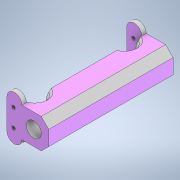
# Autodesk Inventor part: rollerbase(v2)
Saved by Autodesk Inventor 2022 (Build 260153000, 153)
## iProperties
Created: 2022-10-27
Part Number: rollerbase(v2)
Material: Generic
Document SubType Name: Modeling
Designer: matia
Density: 1 g/cm^3
Appearance: Default
Author: matia
Autodesk Inventor part; units mm, degrees
ref_plane "YZ Plane" through (0, 0, 0) normal (1, 0, 0) x (0, 1, 0)
ref_plane "XZ Plane" through (0, 0, 0) normal (0, 1, 0) x (-1, 0, 0)
ref_plane "XY Plane" through (0, 0, 0) normal (0, 0, 1) x (1, 0, 0)
sketch "Sketch1" plane through (0, 0, 0) normal (0, 1, 0) x (-1, 0, 0)
  line L0 (0, -3.556) -> (0, -34.544)
  arc A0 (0, 3.556) -> (0, -3.556) centre (0, 0) ccw
  arc A1 (0, -34.544) -> (0, -41.656) centre (0, -38.1) ccw
  line L1 (0, 3.556) -> (0, 5.461)
  line L2 (0, -41.656) -> (0, -43.561)
  line L3 (0, 7.366) -> (-13.335, 7.366)
  line L4 (0, -45.466) -> (-13.335, -45.466)
  line L5 (-13.335, -45.466) -> (-13.335, 7.366)
  line L6 (0, 7.366) -> (3.175, 7.366)
  line L7 (3.175, 5.461) -> (0, 5.461)
  line L8 (0, -45.466) -> (3.175, -45.466)
  line L9 (3.175, -43.561) -> (0, -43.561)
  line L10 (3.175, 7.366) -> (4.445, 7.366)
  line L11 (4.445, 7.366) -> (4.445, 5.461)
  line L12 (4.445, 5.461) -> (3.175, 5.461)
  line L13 (3.175, -43.561) -> (4.445, -43.561)
  line L14 (4.445, -43.561) -> (4.445, -45.466)
  line L15 (4.445, -45.466) -> (3.175, -45.466)
  dimension "d1" = 7.112
  constraints: 32 end point, 4 horizontal, 4 perpendicular, 4 point on circle, 3 vertical, 2 centre point, 2 parallel, 2 point on line, 1 coincident
  measures "d1" diameter of A0
extrude "Extrusion1" add sketch "Sketch1" along normal blind 12.7
sketch "Sketch2" plane through (13.335, 0, -45.466) normal (0, 0, -1) x (-1, 0, 0)
  line L0 (13.335, 0) -> (17.78, 0) projected
  line L1 (13.335, 0) -> (15.5575, 0)
  line L2 (17.78, 0) -> (17.78, 12.7) projected
  line L3 (17.78, 6.35) -> (15.5575, 6.35)
  line L4 (15.5575, 6.35) -> (15.5575, 0)
  line L5 (15.5575, 6.35) -> (15.5575, 3.81)
  circle A0 centre (15.5575, 3.81) radius 1.5875
  line L6 (15.5575, 6.35) -> (15.5575, 8.89)
  circle A1 centre (15.5575, 8.89) radius 1.5875
  dimension "d10" = 2.54
  dimension "d11" = 3.175
  dimension "d12" = 2.54
  dimension "d13" = 3.175
  constraints: 10 end point, 2 centre point, 2 coincident, 2 midpoint, 1 horizontal, 1 perpendicular, 1 point on line, 1 vertical
  measures "d10" distance of L3.end L5.end
  measures "d11" diameter of A0
  measures "d12" distance of L3.end L6.end
  measures "d13" diameter of A1
extrude "Extrusion2" cut sketch "Sketch2" against normal through all contours A0 L4 | L4 A0 | A1
sketch "Sketch3" plane through (0, 12.7, 0) normal (0, 1, 0) x (1, 0, 0)
  line L0 (0, -5.461) -> (1.905, -5.461)
  line L1 (1.905, -5.461) -> (1.905, 43.561)
  line L2 (1.905, 43.561) -> (0, 43.561)
  line L3 (0, 43.561) -> (0, -5.461)
  point P0 (0, 0)
  dimension "d16" = 1.905
  constraints: 8 end point, 2 parallel, 1 horizontal, 1 perpendicular
  measures "d16" distance of L2.end L1.end
extrude "Extrusion3" cut sketch "Sketch3" against normal through all
chamfer "Chamfer1" distance 3.175 angle 45 2 edges at (13.335, 12.7, -19.05) (13.335, 0, -19.05)
chamfer "Chamfer2" distance 1.905 angle 45 4 edges at (3.556, 0, -38.1) (3.556, 0, 0) (3.556, 12.7, 0) (3.556, 12.7, -38.1)
fillet "Fillet1" radius 3.175 4 edges at (3.556, 1.905, -38.1) (3.556, 10.795, -38.1) (3.556, 1.905, 0) (3.556, 10.795, 0)
sketch "Sketch4" plane through (-4.445, 0, 7.366) normal (0, 0, 1) x (1, 0, 0)
  line L0 (17.78, 3.175) -> (17.78, 9.525) projected
  line L1 (17.78, 6.35) -> (10.16, 6.35)
  line L2 (17.78, 6.35) -> (11.43, 6.35)
  circle A0 centre (11.43, 6.35) radius 3.175
  point P0 (4.445, 0)
  dimension "d26" = 7.62
  dimension "d27" = 6.35
  dimension "d28" = 6.35
  constraints: 4 end point, 1 centre point, 1 coincident, 1 horizontal, 1 midpoint, 1 point on line
  measures "d26" distance of L1.start L1.end
  measures "d27" distance of L1.start L2.end
  measures "d28" diameter of A0
extrude "Extrusion4" cut sketch "Sketch4" against normal blind 12.7
sketch "Sketch5" plane through (-4.445, 0, -45.466) normal (0, 0, -1) x (-1, 0, 0)
  line L0 (-17.78, 3.175) -> (-17.78, 9.525) projected
  line L1 (-17.78, 6.35) -> (-11.43, 6.35)
  circle A0 centre (-11.43, 6.35) radius 3.175
  point P0 (-4.445, 0)
  dimension "d31" = 6.35
  constraints: 2 end point, 1 centre point, 1 coincident, 1 horizontal, 1 midpoint
  measures "d31" distance of L1.start L1.end
extrude "Extrusion5" cut sketch "Sketch5" against normal blind 12.7
sketch "Sketch6" plane through (-4.445, 0, -43.561) normal (0, 0, 1) x (1, 0, 0)
  line L0 (0, 12.7) -> (6.35, 12.7) projected
  line L1 (6.35, 12.7) -> (6.35, 0)
  line L2 (0, 0) -> (6.35, 0) projected
  line L3 (6.35, 0) -> (0, 0)
  line L4 (0, 0) -> (0, 12.7)
  point P0 (4.445, 0)
  constraints: 6 end point, 2 perpendicular, 1 vertical
sketch "Sketch7" plane through (0, 12.7, 0) normal (0, 1, 0) x (1, 0, 0)
  line L0 (-4.445, 43.561) -> (1.905, 43.561) projected
  line L1 (-4.445, 45.466) -> (-4.445, 43.561) projected
  line L2 (-4.445, 43.561) -> (-4.445, 45.466)
  line L3 (-4.445, 43.561) -> (1.905, 43.561)
  line L4 (10.16, 45.466) -> (-4.445, 45.466) projected
  line L5 (1.905, 45.466) -> (1.905, 43.561)
  line L6 (1.905, 45.466) -> (-4.445, 45.466)
  line L7 (-3.81, 45.466) -> (-0.635, 45.466) projected
  point P0 (0, 0)
  constraints: 8 end point, 3 collinear, 1 perpendicular, 1 point on line
extrude "Extrusion6" add sketch "Sketch7" along normal blind 3.175
sketch "Sketch8" plane through (0, 0, 0) normal (0, -1, 0) x (1, 0, 0)
  line L0 (1.905, -45.466) -> (1.905, -43.561) projected
  line L1 (1.905, -43.561) -> (1.905, -45.466)
  line L2 (10.16, -45.466) -> (-4.445, -45.466) projected
  line L3 (1.905, -45.466) -> (-4.445, -45.466)
  line L4 (-4.445, -43.561) -> (1.905, -43.561) projected
  line L5 (-4.445, -45.466) -> (-4.445, -43.561)
  point P0 (0, 0)
  constraints: 6 end point, 2 perpendicular, 1 collinear
extrude "Extrusion7" add sketch "Sketch8" along normal blind 3.175
sketch "Sketch9" plane through (0, 0, 0) normal (0, -1, 0) x (1, 0, 0)
  point P0 (0, 0)
ref_plane "Work Plane1" through (13.335, 3.175, -19.05) normal (0, 0, -1) x (-1, 0, 0)
mirror "Mirror1" about plane through (13.335, 3.175, -19.05) normal (0, 0, -1) of "Extrusion3", "Fillet1", "Chamfer2", "Extrusion7", "Extrusion1", "Extrusion6", "Extrusion5", "Extrusion2", "Chamfer1"
sketch "Sketch10" plane through (1.905, 0, 7.366) normal (0, 0, 1) x (1, 0, 0)
  circle A0 centre (-4.1275, 8.89) radius 1.5875 projected
  circle A1 centre (-4.1275, 8.89) radius 1.5875
  circle A2 centre (-4.1275, 3.81) radius 1.5875 projected
  circle A3 centre (-4.1275, 3.81) radius 1.5875
  point P0 (-1.905, 0)
  constraints: 2 centre point, 2 coincident
extrude "Extrusion8" add sketch "Sketch10" against normal blind 1.905
sketch "Sketch11" plane through (1.905, 0, 7.366) normal (0, 0, 1) x (1, 0, 0)
  line L0 (-6.35, -3.175) -> (-6.35, 15.875) projected
  line L1 (-6.35, 6.35) -> (-3.4925, 6.35)
  line L2 (-3.4925, 6.35) -> (-3.4925, 10.16)
  line L3 (-3.4925, 10.16) -> (-3.4925, 2.54)
  circle A0 centre (-3.4925, 2.54) radius 1.5875
  circle A1 centre (-3.4925, 10.16) radius 1.5875
  point P0 (-1.905, 0)
  dimension "d41" = 2.8575
  dimension "d42" = 3.81
  dimension "d43" = 7.62
  dimension "d44" = 3.175
  dimension "d45" = 3.175
  constraints: 6 end point, 2 centre point, 2 coincident, 1 horizontal, 1 midpoint, 1 point on line, 1 vertical
  measures "d41" distance of L1.start L1.end
  measures "d42" distance of L1.end L2.end
  measures "d43" distance of L2.end L3.end
  measures "d44" diameter of A0
  measures "d45" diameter of A1
hole "Hole1" at (-1.5875, 10.16, 7.366) direction (0, 0, -1) diameter 1.4249 depth 1.905 thread size "1-64 UNC" class "2B" standard "ANSI Unified Screw Threads"
hole "Hole2" at (-1.5875, 2.54, 7.366) direction (0, 0, -1) diameter 1.4249 depth 1.905 thread size "1-64 UNC" class "2B" standard "ANSI Unified Screw Threads"
sketch "Sketch12" plane through (1.905, 15.875, -45.466) normal (0, 0, -1) x (-1, 0, 0)
  circle A0 centre (4.1275, -12.065) radius 1.5875 projected
  circle A1 centre (4.1275, -12.065) radius 1.5875
  circle A2 centre (4.1275, -6.985) radius 1.5875 projected
  circle A3 centre (4.1275, -6.985) radius 1.5875
  point P0 (1.905, -15.875)
  constraints: 2 centre point, 2 coincident
extrude "Extrusion9" add sketch "Sketch12" against normal blind 1.905
sketch "Sketch13" plane through (1.905, 15.875, -45.466) normal (0, 0, -1) x (-1, 0, 0)
  line L0 (6.35, -19.05) -> (6.35, 0) projected
  line L1 (6.35, -9.525) -> (3.4925, -9.525)
  circle A0 centre (3.4925, -13.335) radius 0.7125 projected
  line L2 (3.4925, -9.525) -> (3.4925, -13.335)
  circle A1 centre (3.4925, -5.715) radius 0.7125 projected
  line L3 (3.4925, -13.335) -> (3.4925, -5.715)
  circle A2 centre (3.4925, -13.335) radius 0.7125
  circle A3 centre (3.4925, -5.715) radius 0.7125
  point P0 (1.905, -15.875)
  dimension "d62" = 2.8575
  constraints: 6 end point, 2 centre point, 2 coincident, 2 concentric, 1 horizontal, 1 midpoint
  measures "d62" distance of L1.start L1.end
hole "Hole3" at (-1.5875, 2.54, -45.466) direction (0, 0, 1) diameter 1.4249 depth 1.905 thread size "1-64 UNC" class "2B" standard "ANSI Unified Screw Threads"
hole "Hole4" at (-1.5875, 10.16, -45.466) direction (0, 0, 1) diameter 1.4249 depth 1.905 thread size "1-64 UNC" class "2B" standard "ANSI Unified Screw Threads"
fillet "Fillet2" radius 3.175 8 edges at (-4.445, 15.875, 6.4135) (1.905, 15.875, 6.4135) (-4.445, -3.175, 6.4135) (-4.445, -3.175, -44.5135) (-4.445, 15.875, -44.5135) (1.905, 15.875, -44.5135) (1.905, -3.175, -44.5135) (1.905, -3.175, 6.4135)
body "Solid1"
